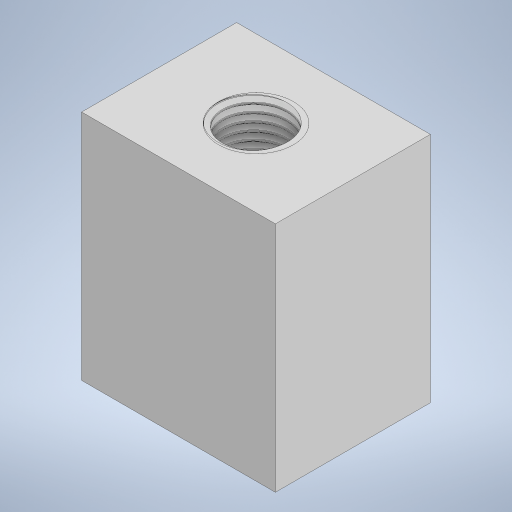
# Autodesk Inventor part: Tensile_test_bottom_adapter_short
Saved by Autodesk Inventor 2024 (Build 280153000, 153)
## iProperties
Created: 2023-09-15
Part Number: Tensile_test_bottom_adapter_short
Material: 일반
Document SubType Name: Modeling
Designer: jsw
Density: 1 g/cm^3
Appearance: 기본값
Author: jsw
Autodesk Inventor part; units mm, degrees
ref_plane "YZ Plane" through (0, 0, 0) normal (1, 0, 0) x (0, 1, 0)
ref_plane "XZ Plane" through (0, 0, 0) normal (0, 1, 0) x (-1, 0, 0)
ref_plane "XY Plane" through (0, 0, 0) normal (0, 0, 1) x (1, 0, 0)
sketch "스케치1" plane through (0, 0, 0) normal (0, 1, 0) x (-1, 0, 0)
  line L0 (-12.5, 10) -> (12.5, 10)
  line L1 (12.5, 10) -> (12.5, -10)
  line L2 (12.5, -10) -> (-12.5, -10)
  line L3 (-12.5, -10) -> (-12.5, 10)
  line L4 (-12.5, 10) -> (12.5, -10) construction
  line L5 (12.5, 10) -> (-12.5, -10) construction
  circle A0 centre (0, 0) radius 8
  dimension "d0" = 25
  dimension "d1" = 20
  dimension "d2" = 16
  constraints: 12 end point, 2 midpoint, 2 parallel, 1 centre point, 1 coincident, 1 horizontal, 1 perpendicular
  measures "d0" distance of L1.end L2.end
  measures "d1" distance of L0.end L1.end
  measures "d2" diameter of A0
extrude "돌출1" add sketch "스케치1" along normal blind 10
sketch "스케치3" plane through (0, 10, 0) normal (0, 1, 0) x (1, 0, 0)
  line L0 (12.5, 10) -> (-12.5, 10) projected
  line L1 (-12.5, 10) -> (-12.5, -10) projected
  line L2 (-12.5, -10) -> (12.5, -10) projected
  line L3 (12.5, -10) -> (12.5, 10) projected
  circle A0 centre (0, 0) radius 8 projected
extrude "돌출3" add sketch "스케치3" along normal blind 20 contours L3 L2 L1 L0 | A0
sketch "스케치6" plane through (0, 30, 0) normal (0, 1, 0) x (1, 0, 0)
  circle A0 centre (0, 0) radius 4.826
  dimension "d20" = 9.652
  constraints: 1 centre point, 1 coincident
  measures "d20" diameter of A0
extrude "돌출6" cut sketch "스케치6" against normal blind 7.62
thread "스레드15" size "0.390-27 UNS" class "2B" standard "ANSI Unified Screw Threads" full length
sketch "스케치32" plane through (0, 22.38, 0) normal (-1, 0, 0) x (0, 0, 1)
  line L0 (4.826, 0) -> (4.826, 7.62)
  line L1 (4.826, 7.62) -> (4.1285, 7.62)
  line L2 (4.1285, 7.62) -> (4.1285, 0)
  line L3 (4.1285, 0) -> (4.826, 0)
  line L4 (0, -28.38) -> (0, 13.62) projected
  constraints: 8 end point
revolve "회전13" add sketch "스케치32" angle 360 about axis through (0, 22.38, 0) along (0, 1, 0) separate body
sketch "스케치31" plane through (0, 22.38, 4.826) normal (1, 0, 0) x (0, 1, 0)
  line L0 (-0.5489, -0.0477) -> (-0.4705, -0.0477) construction
  line L1 (0.0783, -0.6501) -> (-0.0001, -0.8007) construction
  line L2 (-0.9408, -0.8007) -> (-1.0192, -0.6501) construction
  line L3 (-0.3921, -0.0477) -> (-0.4705, 0.1029) construction
  line L4 (-0.4705, 0.1029) -> (-0.5489, -0.0477) construction
  line L5 (-0.9408, -0.8007) -> (-0.8624, -0.6501) construction
  line L6 (-0.3921, -0.0477) -> (-0.0785, -0.6501)
  line L7 (-1.0192, -0.6501) -> (-0.8624, -0.6501) construction
  arc A0 (-1.0192, -0.6501) -> (-0.9408, -0.6977) centre (-0.9408, -0.6093) ccw construction
  line L8 (0.0783, -0.6501) -> (-0.0785, -0.6501) construction
  line L9 (-0.9408, -0.8007) -> (-0.9408, -0.6501) construction
  line L10 (-0.0001, -0.8007) -> (-0.0001, -0.6501) construction
  line L11 (-0.4705, 0.1029) -> (-0.4705, -0.0002) construction
  line L12 (-0.9408, -0.6977) -> (-0.0001, -0.6977)
  arc A1 (-0.9408, -0.6977) -> (-0.8624, -0.6501) centre (-0.9408, -0.6093) ccw
  line L13 (-0.0785, -0.6501) -> (-0.0001, -0.8007) construction
  line L14 (-0.8624, -0.6501) -> (-0.5489, -0.0477)
  line L15 (-0.0001, -0.0002) -> (-0.0001, 0.0177)
  line L16 (-0.0001, 0.0177) -> (-0.0001, -0.0002)
  line L17 (-0.0001, -0.0002) -> (0.0334, -0.0002)
  arc A2 (-0.0785, -0.6501) -> (-0.0001, -0.6977) centre (-0.0001, -0.6093) ccw
  arc A3 (-0.0001, -0.6977) -> (0.0783, -0.6501) centre (-0.0001, -0.6093) ccw construction
  arc A4 (-0.4705, -0.0002) -> (-0.5489, -0.0477) centre (-0.4705, -0.0886) ccw
  arc A5 (-0.3921, -0.0477) -> (-0.4705, -0.0002) centre (-0.4705, -0.0886) ccw
  line L18 (-0.4705, -0.0002) -> (-0.4705, -0.0477) construction
  line L19 (-0.4705, -0.0477) -> (-0.3921, -0.0477) construction
  dimension "d269" = 55
  dimension "d270" = 0.1506
  dimension "d271" = 0.1506
  dimension "d274" = 0.9407
  constraints: 40 end point, 12 point on circle, 10 parallel, 9 tangent, 7 collinear, 6 centre point, 2 midpoint, 2 point on line, 1 horizontal, 1 perpendicular, 4 other
  measures "d269" angle of L6 L14
  measures "d270" distance of L3.end L0.end
  measures "d271" distance of L1.end L10.end
  measures "d274" distance from line of L1.end L9
coil "코일13" sketch "스케치31" operation cut axis through (0, 22.38, 0) along (0, 1, 0) pitch 1.0348 turns 9.181818 hand right bodies 2
equation "\"d269\" = d276"
equation "\"d34\" = 55deg"
equation "\"d54\" = 55deg"
equation "\"d74\" = 55deg"
equation "\"d94\" = 55deg"
equation "\"d116\" = 55deg"
equation "\"d136\" = 55deg"
equation "\"d156\" = 55deg"
equation "\"d176\" = 55deg"
equation "\"d196\" = 55deg"
equation "\"d216\" = 55deg"
equation "\"d236\" = 55deg"
equation "\"d256\" = 55deg"
equation "\"d276\" = 55deg"
